Autodesk Inventor part; units mm, degrees
(part 2 of 2)
  arc A124 (91, -280.3541) -> (93.3541, -278) centre (90, -277) ccw
  line L172 (89, -298) -> (68.2, -298)
  line L173 (121.8, -298) -> (101, -298)
  line L174 (99, -298) -> (91, -298)
  line L175 (152.4442, -54.0809) -> (152.4442, -2)
  line L176 (150.4442, -54.0809) -> (150.4442, -2)
  line L177 (149.6145, -54.4513) -> (135.1648, -41.4947)
  line L178 (148.2793, -55.9404) -> (133.8296, -42.9837)
  arc A125 (148.2793, -55.9404) -> (152.4442, -54.0809) centre (151.4442, -57.435) ccw
  arc A126 (150.4442, -54.0809) -> (149.6145, -54.4513) centre (151.4442, -57.435) ccw
  line L179 (99, -2) -> (91, -2)
  line L180 (89, -2) -> (68.2, -2)
  point P0 (0, 0)
  dimension "d490" = 2
  dimension "d496" = 2
  dimension "d505" = 2
  dimension "d513" = 2
  dimension "d562" = 2
  constraints: 300 end point, 176 point on circle, 85 centre point, 22 parallel, 6 perpendicular, 1 point on line
  measures "d490" distance between parallel lines of L21 L33
  measures "d496" distance between parallel lines of L5 L38
  measures "d505" distance between parallel lines of L13 L45
  measures "d513" distance between parallel lines of L3 L51
  measures "d562" distance between parallel lines of L22 L54
extrude "돌출28" cut sketch "스케치29" against normal blind 3.3 contours A79 L92 A76 L36 L95 L31 | L32 A65 L71 A59 L68 A58 L38 A53 L66 A50 L64 L75 L73 A61 L78 A63 L77 L53 | L33 L173 L167 A121 L170 L168 L83 A69 L82 A68 | L34 A77 L90 A73 L88 L169 L171 A123 L164 L172 | L35 A75 L93 A80 L94 L96 L97 L100 A81 L98 L106 A83 L109 A87 L110 L89 A74 L91 A78 | L37 A57 L69 A60 L70 A66 L54 A67 L81 A70 L84 L87 A71 L85 A56 | L39 A51 L112 A91 L113 A49 L67 A54 | L40 A55 L86 A72 L115 A90 L111 A52 | L56 L176 A126 L177 A45 L41 | A44 L178 A125 L175 L55 L57 L58 A47 L61 L65 A48 L114 A89 L150 L155 A116 L158 A43 L42 | A42 L157 A115 L156 L149 L146 A112 L144 L145 L43 | L180 L141 A113 L147 L148 L152 A118 L153 A106 L44 | L45 A103 L129 A101 L124 L135 L132 A107 L138 A109 L136 L130 | L46 A105 L154 A117 L151 L161 A119 L159 A93 L48 A94 L127 A100 L128 A104 | L47 L134 L131 L137 A110 L139 A108 | A92 L160 A120 L162 A88 L117 A99 L49 | A98 L119 A86 L108 A84 L121 A97 L50 | A96 L123 A85 L105 L133 L125 A102 L126 A95 L51 | L52 L76 A64 L79 A62 L72 L74 | L59 L62 L63 L60 A46 | A82 L101 L102 L103 L99 | L140 L179 L143 A111 L142 A114 | A124 L165 A122 L166 L174 L163
sketch "스케치30" plane through (0, 4, 0) normal (0, 1, 0) x (1, 0, 0)
  line L0 (229, -260) -> (229, -300) projected
  line L1 (229, -300) -> (230, -300) projected
  line L2 (230, -300) -> (230, -260) projected
  line L3 (230, -260) -> (229, -260) projected
  line L4 (229, 0) -> (229, -40) projected
  line L5 (229, -40) -> (230, -40) projected
  line L6 (230, -40) -> (230, 0) projected
  line L7 (230, 0) -> (229, 0) projected
  line L8 (-39, -40) -> (-39, 0) projected
  line L9 (-39, 0) -> (-40, 0) projected
  line L10 (-40, 0) -> (-40, -40) projected
  line L11 (-40, -40) -> (-39, -40) projected
  line L12 (-39, -300) -> (-39, -260) projected
  line L13 (-39, -260) -> (-40, -260) projected
  line L14 (-40, -260) -> (-40, -300) projected
  line L15 (-40, -300) -> (-39, -300) projected
  line L16 (230, -300) -> (230, -260) projected
  line L17 (230, -300) -> (190, -300)
  line L18 (190, -300) -> (190, -260)
  line L19 (190, -260) -> (230, -260)
  line L20 (230, -260) -> (230, -300)
  line L21 (230, 0) -> (229, 0) projected
  line L22 (230, 0) -> (190, 0)
  line L23 (190, 0) -> (190, -40)
  line L24 (190, -40) -> (230, -40)
  line L25 (230, -40) -> (230, 0)
  line L26 (-40, 0) -> (0, 0)
  line L27 (0, 0) -> (0, -40)
  line L28 (0, -40) -> (-40, -40)
  line L29 (-40, -40) -> (-40, 0)
  line L30 (-40, -300) -> (0, -300)
  line L31 (0, -300) -> (0, -260)
  line L32 (0, -260) -> (-40, -260)
  line L33 (-40, -260) -> (-40, -300)
  point P0 (0, 0)
  constraints: 32 end point, 8 parallel, 4 horizontal, 4 perpendicular
extrude "돌출29" cut sketch "스케치30" against normal blind 10
